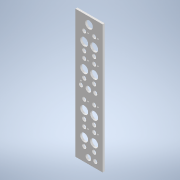
# Autodesk Inventor part: HalfInterlockBox
Saved by Autodesk Inventor 2020 (Build 240168000, 168)
## iProperties
Created: 2019-09-04
Part Number: HalfInterlockBox
Material: Generic
Document SubType Name: Modeling
Designer: Eric
Density: 1 g/cm^3
Appearance: Default
Author: Eric
Autodesk Inventor part; units mm, degrees
ref_plane "YZ Plane" through (0, 0, 0) normal (1, 0, 0) x (0, 1, 0)
ref_plane "XZ Plane" through (0, 0, 0) normal (0, 1, 0) x (-1, 0, 0)
sketch "Sketch1" plane through (0, 0, 0) normal (0, 0, 1) x (1, 0, 0)
  line L0 (-43.688, 0) -> (-43.688, 415.3) projected
  line L1 (0, 0) -> (0, 415.3) projected
  circle A0 centre (-7.6009, 150.0066) radius 1.1 projected
  circle A1 centre (-13.6588, 173.1577) radius 6.4135 projected
  circle A2 centre (-13.6588, 134.9467) radius 6.4135 projected
  circle A3 centre (-7.6009, 188.2176) radius 1.1 projected
  circle A4 centre (-7.6009, 92.9676) radius 1.1 projected
  circle A5 centre (-13.6588, 245.4367) radius 6.4135 projected
  circle A6 centre (-13.6588, 77.9077) radius 6.4135 projected
  circle A7 centre (-7.6009, 260.4966) radius 1.1 projected
  circle A8 centre (-7.6009, 54.7566) radius 1.1 projected
  circle A9 centre (-13.6588, 283.6477) radius 6.4135 projected
  circle A10 centre (-13.6588, 39.6967) radius 6.4135 projected
  circle A11 centre (-7.6009, 298.7076) radius 1.1 projected
  line L2 (-7.3698, 0) -> (-7.3698, 12.7) projected
  line L3 (-7.3698, 0) -> (-36.3182, 0) projected
  line L4 (-36.3182, 0) -> (-36.3182, 12.7) projected
  line L5 (-36.3182, 12.7) -> (-39.4462, 12.7) projected
  line L6 (-39.4462, 12.7) -> (-39.4462, 402.6) projected
  line L7 (-39.4462, 402.6) -> (-36.3182, 402.6) projected
  line L8 (-36.3182, 402.6) -> (-36.3182, 415.3) projected
  line L9 (-36.3182, 415.3) -> (-7.3698, 415.3) projected
  line L10 (-7.3698, 402.6) -> (-7.3698, 415.3) projected
  line L11 (-7.3698, 402.6) -> (-4.2418, 402.6) projected
  line L12 (-4.2418, 402.6) -> (-4.2418, 12.7) projected
  line L13 (-4.2418, 12.7) -> (-7.3698, 12.7) projected
  circle A12 centre (-13.6588, 340.6867) radius 6.4135 projected
  circle A13 centre (-7.6009, 355.7466) radius 1.1 projected
  circle A14 centre (-13.6588, 378.8977) radius 6.4135 projected
  circle A15 centre (-34.9052, 110.3753) radius 3.2004 projected
  circle A16 centre (-34.9052, 316.1153) radius 3.2004 projected
  circle A17 centre (-7.6009, 393.9576) radius 1.1 projected
  circle A18 centre (-11.9075, 15.1253) radius 3.302 projected
  circle A19 centre (-23.6029, 54.7566) radius 1.1 projected
  circle A20 centre (-23.6029, 92.9676) radius 1.1 projected
  circle A21 centre (-23.6029, 188.2176) radius 1.1 projected
  circle A22 centre (-23.6029, 260.4966) radius 1.1 projected
  circle A23 centre (-34.9052, 322.1732) radius 1.1 projected
  circle A24 centre (-23.6029, 355.7466) radius 1.1 projected
  circle A25 centre (-23.6029, 393.9576) radius 1.1 projected
  circle A26 centre (-23.6029, 298.7076) radius 1.1 projected
  circle A27 centre (-23.6029, 150.0066) radius 1.1 projected
  circle A28 centre (-34.9052, 116.4332) radius 1.1 projected
  circle A29 centre (-11.9075, 316.1153) radius 3.302 projected
  circle A30 centre (-13.6588, 328.1211) radius 3.302 projected
  circle A31 centre (-13.6588, 366.3321) radius 3.302 projected
  circle A32 centre (-13.6588, 271.0821) radius 3.302 projected
  circle A33 centre (-13.6588, 232.8711) radius 3.302 projected
  circle A34 centre (-29.6608, 160.5921) radius 3.302 projected
  circle A35 centre (-29.6608, 122.3811) radius 3.302 projected
  circle A36 centre (-11.9075, 110.3753) radius 3.302 projected
  circle A37 centre (-13.6588, 65.3421) radius 3.302 projected
  circle A38 centre (-13.6588, 27.1311) radius 3.302 projected
  circle A39 centre (-29.6608, 27.1311) radius 3.302 projected
  circle A40 centre (-29.6608, 65.3421) radius 3.302 projected
  circle A41 centre (-13.6588, 122.3811) radius 3.302 projected
  circle A42 centre (-13.6588, 160.5921) radius 3.302 projected
  circle A43 centre (-11.9075, 220.8653) radius 3.302 projected
  circle A44 centre (-29.6608, 232.8711) radius 3.302 projected
  circle A45 centre (-29.6608, 271.0821) radius 3.302 projected
  circle A46 centre (-29.6608, 366.3321) radius 3.302 projected
  circle A47 centre (-29.6608, 328.1211) radius 3.302 projected
  circle A48 centre (-29.6583, 340.6867) radius 6.4135 projected
  circle A49 centre (-29.6583, 378.8977) radius 6.4135 projected
  circle A50 centre (-29.6583, 245.4367) radius 6.4135 projected
  circle A51 centre (-29.6583, 173.1577) radius 6.4135 projected
  circle A52 centre (-29.6583, 134.9467) radius 6.4135 projected
  circle A53 centre (-29.6583, 39.6967) radius 6.4135 projected
  circle A54 centre (-29.6583, 77.9077) radius 6.4135 projected
  circle A55 centre (-29.6583, 283.6477) radius 6.4135 projected
  circle A56 centre (-22.9108, 110.3753) radius 4.5 projected
  circle A57 centre (-22.9108, 220.8653) radius 4.5 projected
  circle A58 centre (-22.9108, 316.1153) radius 4.5 projected
  circle A59 centre (-13.6588, 355.7466) radius 3.2004 projected
  circle A60 centre (-29.6608, 393.9576) radius 3.2004 projected
  circle A61 centre (-29.6608, 298.7076) radius 3.2004 projected
  circle A62 centre (-13.6588, 260.4966) radius 3.2004 projected
  circle A63 centre (-13.6588, 188.2176) radius 3.2004 projected
  circle A64 centre (-13.6588, 150.0066) radius 3.2004 projected
  circle A65 centre (-13.6588, 92.9676) radius 3.2004 projected
  circle A66 centre (-29.6608, 54.7566) radius 3.2004 projected
  circle A67 centre (-13.6588, 54.7566) radius 3.2004 projected
  circle A68 centre (-29.6608, 92.9676) radius 3.2004 projected
  circle A69 centre (-29.6608, 150.0066) radius 3.2004 projected
  circle A70 centre (-29.6608, 188.2176) radius 3.2004 projected
  circle A71 centre (-29.6608, 260.4966) radius 3.2004 projected
  circle A72 centre (-13.6588, 298.7076) radius 3.2004 projected
  circle A73 centre (-13.6588, 393.9576) radius 3.2004 projected
  circle A74 centre (-29.6608, 355.7466) radius 3.2004 projected
  circle A75 centre (-21.844, 200.6606) radius 6.25 projected
  circle A76 centre (-21.844, 406.4006) radius 6.25 projected
  circle A77 centre (-22.9108, 15.1253) radius 4.5 projected
  line L14 (-36.3182, 0) -> (-43.688, 0)
  line L15 (0, 0) -> (-7.3698, 0)
  line L16 (0, 5.79) -> (-43.688, 5.79)
  line L17 (0, 212.165) -> (-43.688, 212.165)
  dimension "d0" = 206.375
  constraints: 8 end point, 4 point on line, 2 horizontal, 1 collinear, 1 perpendicular
  measures "d0" distance between parallel lines of L16 L17
ref_plane "Work Plane1" through (-39.4462, 0, -3.175) normal (0, 0, -1) x (0, 1, 0)
extrude "Extrusion1" add sketch "Sketch1" against normal up to surface (3.175 mm away) contours L0 L17 L6 L5 L4 L16 | L4 L5 L6 L17 L12 L13 L2 L16 | L2 L13 L12 L17 L1 L16
body "Solid1"
